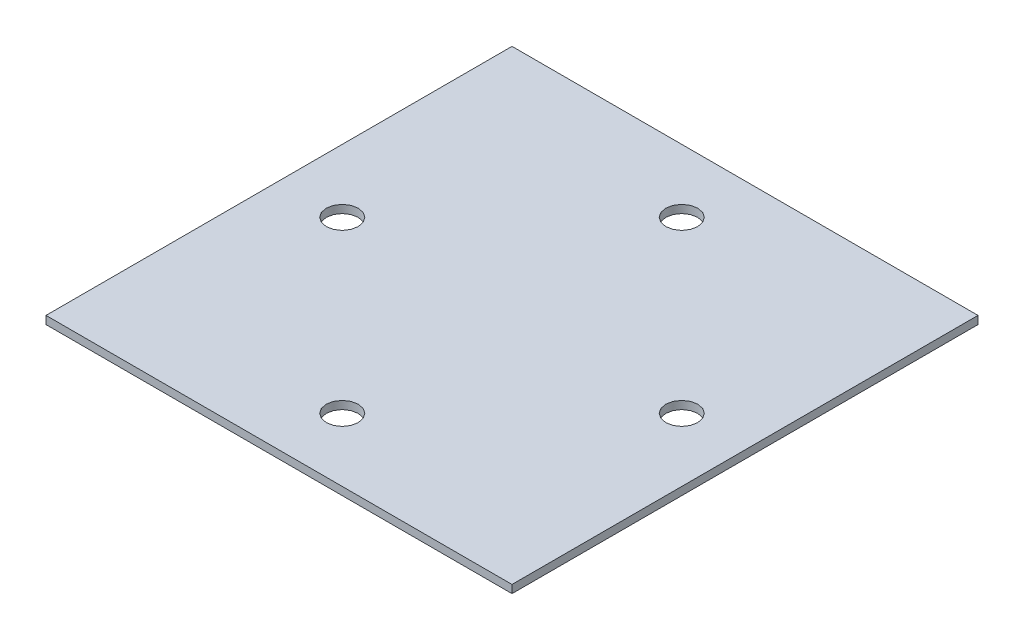
# Autodesk Inventor part: MSC 127 flange frame heel
Saved by Autodesk Inventor 2025 (Build 290162010, 162A)
## iProperties
Created: 2024-07-01
Part Number: MSC 127 flange frame heel
Material: Stainless Steel
Document SubType Name: Sheet Metal
Designer: pokla
Density: 8 g/cm^3
Sheet Metal Rule: AISI304 2mm Die16
Appearance: Default
Author: pokla
Autodesk Inventor part; units mm, degrees
ref_plane "YZ Plane" through (0, 0, 0) normal (1, 0, 0) x (0, 1, 0)
ref_plane "XZ Plane" through (0, 0, 0) normal (0, 1, 0) x (-1, 0, 0)
ref_plane "XY Plane" through (0, 0, 0) normal (0, 0, 1) x (1, 0, 0)
sketch "Sketch1" plane through (0, 0, 0) normal (0, 1, 0) x (-1, 0, 0)
  line L0 (87.5, 87.5) -> (-87.5, 87.5)
  line L1 (-87.5, 87.5) -> (-87.5, -87.5)
  line L2 (-87.5, -87.5) -> (87.5, -87.5)
  line L3 (87.5, -87.5) -> (87.5, 87.5)
  line L4 (87.5, 87.5) -> (-87.5, -87.5) construction
  line L5 (40, 40) -> (-40, 40) construction
  line L6 (-40, 40) -> (-40, -40) construction
  line L7 (-40, -40) -> (40, -40) construction
  line L8 (40, -40) -> (40, 40) construction
  line L9 (-40, 40) -> (40, -40) construction
  point P0 (0, 0)
  point P1 (0, 0)
  point P2 (0, 87.5)
  dimension "d0" = 175
  dimension "d1" = 175
  dimension "d2" = 80
  dimension "d3" = 80
  measures "d0" distance of L2.end L1.end
  measures "d1" distance of L1.end L0.end
  measures "d2" distance of L7.end L6.end
  measures "d3" distance of L6.end L5.end
extrude "Plate1" add sketch "Sketch1" along normal blind 3
sketch "Sketch2" plane through (0, 3, 0) normal (0, 1, 0) x (1, 0, 0)
  circle A0 centre (0, -63.75) radius 6
  line L0 (87.5, -87.5) -> (-87.5, -87.5) projected
  point P0 (0, 0)
  point P1 (0, -87.5)
  dimension "d7" = 23.75
  dimension "d8" = 12
  constraints: 1 centre point, 1 midpoint, 1 vertical alignment
  measures "d7" distance of point (0, -87.5) A0.centre
  measures "d8" diameter of A0
extrude "Extrusion1" cut sketch "Sketch2" against normal blind 10
pattern_circular "Circular Pattern1" count 4 over 360 about axis through (0, -10, 0) along (0, 1, 0) of "Extrusion1"
equation "\"BendReliefWidth\" = Thickness"
equation "\"BendReliefDepth\" = 0.5 * Thickness"
equation "\"CornerReliefSize\" = 4 * Thickness"
equation "\"MinimumRemnant\" = 2 * Thickness"
equation "\"TransitionRadius\" = BendRadius"
equation "\"JacobiRadiusSize\" = BendRadius"
equation "\"GapSize\" = Thickness"
body "Solid1"
